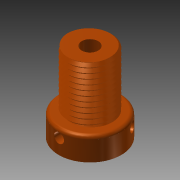
# Autodesk Inventor part: z pulley
Saved by Autodesk Inventor 2013 (Build 170138000, 138)
## iProperties
Created: 2013-09-18
Part Number: z pulley
Material: Generic
Document SubType Name: Modeling
Designer: employee
Density: 1 g/cm^3
Mass: 3.52366 g
Surface Area: 24.1776 cm^2
Volume: 3.52366 cm^3
Author: employee
Autodesk Inventor part; units mm, degrees
ref_plane "YZ Plane" through (0, 0, 0) normal (1, 0, 0) x (0, 1, 0)
ref_plane "XZ Plane" through (0, 0, 0) normal (0, 1, 0) x (-1, 0, 0)
ref_plane "XY Plane" through (0, 0, 0) normal (0, 0, 1) x (1, 0, 0)
sketch "Sketch1" plane through (0, 0, 0) normal (0, 0, 1) x (1, 0, 0)
  circle A0 centre (0, 0) radius 6
  dimension "d0" = 12
  constraints: 1 centre point, 1 coincident
  measures "d0" diameter of A0
extrude "Extrusion1" add sketch "Sketch1" along normal blind 17
sketch "Sketch2" plane through (0, 0, 0) normal (0, 0, -1) x (-1, 0, 0)
  circle A0 centre (0, 0) radius 6 projected
  circle A1 centre (0, 0) radius 9.5
  circle A2 centre (0, 0) radius 2.5
  dimension "d51" = 7
  dimension "d52" = 5
  constraints: 2 centre point, 2 coincident
  measures "d51" radial gap between concentric circles of A1 A2
  measures "d52" diameter of A2
extrude "Extrusion2" add sketch "Sketch2" along normal blind 5 contours A0 | A1 | A2
sketch "Sketch3" plane through (0, 0, 0) normal (0, 1, 0) x (-1, 0, 0)
  line L0 (6, 0) -> (9.5, 0) projected
  line L1 (9.5, 0) -> (9.5, -5) projected
  line L2 (9.5, -5) -> (-9.5, -5) projected
  line L3 (-9.5, -5) -> (-9.5, 0) projected
  line L4 (-9.5, 0) -> (-6, 0) projected
  line L5 (-6, 0) -> (-6, 17) projected
  line L6 (-6, 17) -> (6, 17) projected
  line L7 (6, 17) -> (6, 0) projected
  line L8 (-6, 17) -> (-6, 18.5)
  line L9 (-6, 18.5) -> (-6.75, 17.75)
  line L10 (-6.75, 17.75) -> (-6, 17)
  point P0 (0, 0)
  dimension "d7" = 1.5
  constraints: 6 end point, 2 perpendicular, 1 parallel
  measures "d7" distance of L5.end L8.end
coil "Coil1" sketch "Sketch3" operation add axis through (0, 0, -10) along (0, 0, -1) pitch 1.501 turns 15 hand right contours L10 L9 L8
sketch "Sketch8" plane through (0, 0, -5) normal (0, 0, -1) x (-1, 0, 0)
  circle A0 centre (0, 0) radius 9.5 projected
extrude "Extrusion7" cut sketch "Sketch8" along normal blind 10
sketch "Sketch4" plane through (0, 0, 17) normal (0, 0, 1) x (1, 0, 0)
  arc A0 (5.9999, 0.0251) -> (6, 0) centre (0, 0) ccw projected
  circle A1 centre (0, 0) radius 20
  dimension "d19" = 40
  constraints: 1 centre point, 1 coincident
  measures "d19" diameter of A1
extrude "Extrusion3" cut sketch "Sketch4" along normal through all
sketch "Sketch5" plane through (0, 0, 17) normal (0, 0, 1) x (1, 0, 0)
  arc A0 (6, 0) -> (5.9999, 0.0251) centre (0, 0) ccw projected
  circle A1 centre (0, 0) radius 2.5
  dimension "d23" = 5
  constraints: 1 centre point, 1 coincident
  measures "d23" diameter of A1
extrude "Extrusion4" cut sketch "Sketch5" against normal through all
sketch "Sketch9" plane through (0, 0, 0) normal (0, 1, 0) x (-1, 0, 0)
  circle A0 centre (0, -2.5) radius 1.5
  point P0 (0, 0)
  dimension "d54" = 3
  dimension "d56" = 2.5
  constraints: 1 centre point, 1 vertical alignment
  measures "d54" diameter of A0
  measures "d56" distance of point (0, 0) A0.centre
extrude "Extrusion9" cut sketch "Sketch9" against normal through all
pattern_circular "Circular Pattern1" count 3 over 360 about axis through (0, 0, 0) along (0, 0, -1) of "Extrusion9"
fillet "Fillet1" radius 1 1 edges at (9.5, 0, 0)
sketch "Sketch10" plane through (0, 0, -5) normal (0, 0, -1) x (-1, 0, 0)
  circle A0 centre (0, 0) radius 2.5 projected
  circle A1 centre (0, 0) radius 9.5 projected
extrude "Extrusion10" add sketch "Sketch10" along normal blind 2
body "Solid1"
